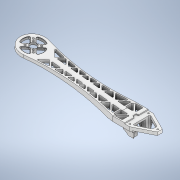
# Autodesk Inventor part: Arm - White
Saved by Autodesk Inventor 2021 (Build 250183000, 183)
## iProperties
Created: 2020-04-25
Part Number: Arm - White
Material: PC/ABS Plastic
Document SubType Name: Modeling
Designer: ljubi
Density: 0.357273 g/cm^3
Appearance: Smooth - White
Author: ljubi
Autodesk Inventor part; units mm, degrees
ref_plane "YZ Plane" through (0, 0, 0) normal (1, 0, 0) x (0, 1, 0)
ref_plane "XZ Plane" through (0, 0, 0) normal (0, 1, 0) x (-1, 0, 0)
ref_plane "XY Plane" through (0, 0, 0) normal (0, 0, 1) x (1, 0, 0)
sketch "Sketch1" plane through (0, 0, 0) normal (0, 1, 0) x (-1, 0, 0)
  line L0 (12, -19) -> (12, 19)
  line L1 (12, 19) -> (0, 19)
  line L2 (0, 19) -> (-30, 4)
  line L3 (-30, 4) -> (-30, -4)
  line L4 (-30, -4) -> (0, -19)
  line L5 (0, -19) -> (12, -19)
  point P0 (0, 0)
  dimension "d0" = 38
  dimension "d1" = 19
  dimension "d2" = 12
  dimension "d3" = 8
  dimension "d4" = 4
  dimension "d5" = 30
  constraints: 12 end point, 2 point on line, 2 vertical alignment, 1 horizontal, 1 parallel, 1 perpendicular, 1 vertical
  measures "d0" distance between parallel lines of L1 L5
  measures "d1" distance from line of L1 point (0, 0)
  measures "d2" distance of L0.end L1.end
  measures "d3" distance of L2.end L3.end
  measures "d4" vertical distance of L2.end point (0, 0)
  measures "d5" distance from line of L3 point (0, 0)
extrude "Extrusion1" add sketch "Sketch1" against normal blind 5
sketch "Sketch2" plane through (0, 0, 0) normal (0, 1, 0) x (1, 0, 0)
  line L0 (0, -19) -> (-12, -19) projected
  line L1 (-12, 19) -> (0, 19) projected
  line L2 (-12, -19) -> (-8, -19)
  line L3 (-8, -19) -> (-8, 19)
  line L4 (-8, 19) -> (-12, 19)
  line L5 (-12, 19) -> (-12, -19)
  point P0 (0, 0)
  dimension "d8" = 8
  constraints: 8 end point, 2 parallel, 1 horizontal, 1 perpendicular, 1 point on line
  measures "d8" distance from line of L3 L1.end
extrude "Extrusion2" add sketch "Sketch2" along normal blind 1.5
sketch "Sketch3" plane through (0, 1.5, 0) normal (0, 1, 0) x (1, 0, 0)
  line L0 (-8, 19) -> (-8, -19) projected
  line L1 (-11.5, -3) -> (-8, -3)
  line L2 (-8, -3) -> (-8, 3)
  line L3 (-8, 3) -> (-11.5, 3)
  line L4 (-11.5, 3) -> (-11.5, -3)
  point P0 (0, 0)
  point P1 (-8, 0)
  dimension "d11" = 6
  dimension "d12" = 3.5
  constraints: 8 end point, 2 midpoint, 2 parallel, 1 horizontal, 1 perpendicular, 1 point on line
  measures "d11" distance between parallel lines of L1 L3
  measures "d12" distance between parallel lines of L4 L0
extrude "Extrusion3" cut sketch "Sketch3" against normal up to surface (1.5 mm away)
fillet "Fillet1" radius 1 4 edges at (-11.5, 0.75, -3) (-11.5, 0.75, 3) (-8, 0.75, 3) (-8, 0.75, -3)
sketch "Sketch4" plane through (0, 0, 0) normal (0, 1, 0) x (1, 0, 0)
  line L0 (30, 4) -> (0, 19) projected
  line L1 (0, -19) -> (30, -4) projected
  line L2 (22, 3.5279) -> (0, 14.5279)
  line L3 (0, -14.5279) -> (22, -3.5279)
  line L4 (22, 3.5279) -> (22, -3.5279)
  line L5 (30, -4) -> (30, 4) projected
  line L6 (0, 14.5279) -> (0, -14.5279)
  point P0 (0, 0)
  dimension "d16" = 4
  dimension "d17" = 4
  dimension "d18" = 8
  constraints: 8 end point, 2 parallel, 2 vertical, 1 point on line
  measures "d16" distance between parallel lines of L1 L3
  measures "d17" distance between parallel lines of L0 L2
  measures "d18" distance between parallel lines of L4 L5
extrude "Extrusion4" cut sketch "Sketch4" against normal through all
fillet "Fillet2" radius 1.5 4 edges at (0, -2.5, -14.5279) (0, -2.5, 14.5279) (22, -2.5, 3.5279) (22, -2.5, -3.5279)
sketch "Sketch5" plane through (-12, -5, -19) normal (-1, 0, 0) x (0, 0, 1)
  line L0 (0, 0) -> (0, 6.5) projected
  line L1 (38, 0) -> (0, 0) projected
  line L2 (38, 6.5) -> (38, 0) projected
  line L3 (0, 6.5) -> (38, 6.5) projected
  point P0 (19, 5)
extrude "Extrusion5" add sketch "Sketch5" along normal blind 15
sketch "Sketch6" plane through (-27, -5, -19) normal (-1, 0, 0) x (0, 0, 1)
  line L0 (0, 0) -> (38, 0)
  line L1 (38, 0) -> (38, -3.5)
  line L2 (38, -3.5) -> (0, -3.5)
  line L3 (0, -3.5) -> (0, 0)
  line L4 (38, 0) -> (38, 6.5) projected
  line L5 (38, 6.5) -> (0, 6.5) projected
  line L6 (0, 6.5) -> (0, 0) projected
  point P0 (19, 5)
  dimension "d24" = 10
  constraints: 8 end point, 2 collinear, 2 parallel, 1 horizontal, 1 perpendicular
  measures "d24" distance between parallel lines of L2 L5
extrude "Extrusion6" add sketch "Sketch6" against normal blind 30 contours L0 L1 L2 L3
sketch "Sketch7" plane through (-8, 0, 19) normal (0, 0, 1) x (1, 0, 0)
  line L0 (11, -8.5) -> (11, -5) projected
  line L1 (11, -8.5) -> (9.2367, -18.5)
  line L2 (9.2367, -18.5) -> (1.2367, -18.5)
  circle A0 centre (-19, -33.9763) radius 25.4763
  line L3 (-19, -8.5) -> (11, -8.5) projected
  line L4 (-19, -8.5) -> (-19, 1.5) projected
  line L5 (0, 1.5) -> (-19, 1.5) projected
  point P0 (8, 0)
  dimension "d27" = 20
  dimension "d28" = 100
  dimension "d29" = 8
  constraints: 4 end point, 1 horizontal, 1 perpendicular, 1 point on line, 3 other
  measures "d27" distance between parallel lines of L2 L5
  measures "d28" angle of L1 L2
  measures "d29" distance of L1.end L2.end
extrude "Extrusion7" add sketch "Sketch7" against normal up to surface (38 mm away) contours L1 L2 A0 L3
sketch "Sketch8" plane through (3, -5, 13.0279) normal (0, 1, 0) x (1, 0, 0)
  line L0 (0, 26.0557) -> (-0.8292, 26.4703) projected
  arc A0 (-0.8292, 26.4703) -> (-3, 25.1287) centre (-1.5, 25.1287) ccw projected
  line L1 (-3, 25.1287) -> (-3, 0.9271) projected
  arc A1 (-3, 0.9271) -> (-0.8292, -0.4146) centre (-1.5, 0.9271) ccw projected
  line L2 (-0.8292, -0.4146) -> (0, 0) projected
  line L3 (0, 26.0557) -> (0, 0) projected
  line L4 (-3, 32.0279) -> (0, 30.5279) projected
  line L5 (0, 32.0279) -> (0, 30.5279) projected
  line L6 (-3, 32.0279) -> (0, 32.0279) projected
  line L7 (0, -4.4721) -> (-3, -5.9721) projected
  line L8 (-3, -5.9721) -> (0, -5.9721) projected
  line L9 (0, -4.4721) -> (0, -5.9721) projected
  point P0 (-3, 13.0279)
extrude "Extrusion8" cut sketch "Sketch8" against normal through all
sketch "Sketch9" plane through (0, 0, 12.1008) normal (1, 0, 0) x (0, 0, -1)
  line L0 (-6.8992, -18.5) -> (31.1008, -18.5) projected
  line L1 (5.6008, -18.5) -> (18.6008, -18.5)
  line L2 (18.6008, -18.5) -> (18.6008, -3)
  line L3 (18.6008, -3) -> (5.6008, -3)
  line L4 (5.6008, -3) -> (5.6008, -18.5)
  line L5 (12.1008, 0) -> (12.1008, -26.1716) construction
  line L6 (16.1008, 0) -> (31.1008, 0) projected
  point P0 (12.1008, -18.5)
  dimension "d34" = 13
  dimension "d35" = 3
  constraints: 10 end point, 2 parallel, 2 point on line, 1 horizontal, 1 midpoint, 1 perpendicular, 1 vertical
  measures "d34" distance between parallel lines of L4 L2
  measures "d35" distance between parallel lines of L6 L3
extrude "Extrusion9" cut sketch "Sketch9" against normal blind 6.5
sketch "Sketch10" plane through (-6.5, 0, 12.1008) normal (1, 0, 0) x (0, 0, -1)
  line L0 (-6.8992, -18.5) -> (31.1008, -18.5) projected
  line L1 (5.6008, -18.5) -> (5.6008, -3) projected
  line L2 (18.6008, -3) -> (18.6008, -18.5) projected
  arc A0 (18.6008, -15) -> (5.6008, -15) centre (12.1008, -15) ccw
  line L3 (-6.8992, 1.5) -> (8.1008, 1.5) projected
  point P0 (12.1008, 0)
  dimension "d38" = 16.5
  constraints: 2 point on circle, 2 point on line, 2 tangent, 1 centre point
  measures "d38" distance from line of A0.centre L3
extrude "Extrusion10" cut sketch "Sketch10" against normal through all
sketch "Sketch11" plane through (-8, 0, 19) normal (0, 0, 1) x (1, 0, 0)
  line L0 (-19, 1.5) -> (-19, -8.5) projected
  line L1 (-19, 1.5) -> (-188.0687, 19.2698)
  line L2 (-188.0687, 19.2698) -> (-188.5914, 14.2972)
  line L3 (0, 1.5) -> (-19, 1.5) projected
  line L4 (-188.5914, 14.2972) -> (-138.8653, 9.0708)
  line L5 (-138.8653, 9.0708) -> (-19, -8.5)
  point P0 (8, 0)
  dimension "d41" = 6
  dimension "d42" = 5
  dimension "d43" = 170
  dimension "d44" = 50
  constraints: 8 end point, 1 parallel, 1 perpendicular
  measures "d41" angle of L1 L3
  measures "d42" distance of L1.end L2.end
  measures "d43" distance of L0.start L1.end
  measures "d44" distance of L2.end L4.end
extrude "Extrusion11" add sketch "Sketch11" against normal up to surface (38 mm away)
sketch "Sketch12" plane through (-196.0687, 19.2698, 19) normal (0.1045285, 0.9945219, 0) x (0.9945219, -0.1045285, 0)
  arc A0 (12.0557, 38) -> (12.0557, 0) centre (21, 19) ccw
  line L0 (197.0089, 6.8992) -> (197.0089, 31.1008) projected
  line L1 (0, 0) -> (0, 38) projected
  line L2 (170, 38) -> (0, 38) projected
  line L3 (170, 0) -> (0, 0) projected
  point P0 (197.0089, 19)
  point P1 (197.0089, 19)
  point P2 (0, 19)
  dimension "d47" = 42
  constraints: 2 point on circle, 2 point on line, 1 centre point, 1 horizontal alignment, 1 midpoint, 1 tangent
  measures "d47" diameter of A0
extrude "Extrusion12" cut sketch "Sketch12" against normal through all
sketch "Sketch13" plane through (-27, 1.5, 19) normal (0.1045285, 0.9945219, 0) x (0.9945219, -0.1045285, 0)
  circle A0 centre (-149, 19) radius 21
  arc A1 (-157.9443, 38) -> (-157.9443, 0) centre (-149, 19) ccw projected
  line L0 (0, 0) -> (-157.9443, 0) projected
  line L1 (0, 38) -> (-157.9443, 38) projected
  point P0 (27.0089, 19)
  point P1 (-140.0557, 38)
  point P2 (-140.0557, 0)
  point P3 (-157.9443, 0)
  constraints: 2 concentric, 1 centre point
extrude "Extrusion13" add sketch "Sketch13" against normal up to surface (5 mm away) contours A0 L1 | L0 A0
sketch "Sketch14" plane through (-27, 1.5, 19) normal (0.1045285, 0.9945219, 0) x (0.9945219, -0.1045285, 0)
  circle A0 centre (-69, -332.0556) radius 339.0556
  arc A1 (-140.0557, 38) -> (-140.0557, 0) centre (-149, 19) ccw projected
  line L0 (-180.4979, 7) -> (84.0441, 7) construction
  line L1 (0, 0) -> (0, 38) projected
  line L2 (0, 0) -> (-140.0557, 0) projected
  point P0 (27.0089, 19)
  point P1 (-137.5403, 0)
  point P2 (-0.4597, 0)
  dimension "d52" = 12
  dimension "d53" = 69
  constraints: 2 end point, 2 tangent, 1 centre point, 1 horizontal
  measures "d52" distance from line of point (27.009, 19) L0
  measures "d53" distance from line of A0.centre L1
extrude "Extrusion14" cut sketch "Sketch14" against normal through all contours L2 A0 picked at (-53.7101, 1.2943)
sketch "Sketch15" plane through (-27, 1.5, 19) normal (0.1045285, 0.9945219, 0) x (0.9945219, -0.1045285, 0)
  circle A0 centre (-69, -332.0556) radius 339.0556
  arc A1 (-0.4597, 0) -> (-137.5403, 0) centre (-69, -332.0556) ccw projected
  line L0 (-137.5403, 0) -> (-140.0557, 0) projected
  arc A2 (-140.0557, 38) -> (-140.0557, 0) centre (-149, 19) ccw projected
  point P0 (27.0089, 19)
  point P1 (-144.3341, -1.4751)
  point P2 (-137.5403, 0)
  constraints: 2 concentric, 1 centre point
extrude "Extrusion15" add sketch "Sketch15" against normal up to surface (5 mm away) contours A2 L0 A0
mirror "Mirror1" about plane through (0, 0, 0) normal (0, 0, 1) of "Extrusion14", "Extrusion15"
sketch "Sketch16" plane through (-27, 1.5, 19) normal (0.1045285, 0.9945219, 0) x (0.9945219, -0.1045285, 0)
  circle A0 centre (-149, 19) radius 5.5
  arc A1 (-144.3341, 39.4751) -> (-144.3341, -1.4751) centre (-149, 19) ccw projected
  point P0 (27.0089, 19)
  dimension "d58" = 11
  constraints: 1 centre point, 1 concentric
  measures "d58" diameter of A0
extrude "Extrusion16" cut sketch "Sketch16" against normal through all
sketch "Sketch17" plane through (-27, 1.5, 19) normal (0.1045285, 0.9945219, 0) x (0.9945219, -0.1045285, 0)
  circle A0 centre (-149, 19) radius 5.5 projected
  line L0 (-149, 19) -> (-171.99, -3.99) construction
  line L1 (-149, 19) -> (-149, -8.9855) construction
  line L2 (-149, 19) -> (-175.0574, 45.0574) construction
  line L3 (-161.209, 12.0943) -> (-155.364, 17.9393)
  line L4 (-161.209, 25.9057) -> (-155.364, 20.0607)
  arc A1 (-144.3341, 39.4751) -> (-144.3341, -1.4751) centre (-149, 19) ccw projected
  arc A2 (-163.6424, 25.4497) -> (-163.6424, 12.5503) centre (-149, 19) ccw
  arc A3 (-155.364, 17.9393) -> (-155.364, 20.0607) centre (-156.4246, 19) ccw
  arc A4 (-161.209, 25.9057) -> (-163.6424, 25.4497) centre (-162.2697, 24.8451) ccw
  arc A5 (-163.6424, 12.5503) -> (-161.209, 12.0943) centre (-162.2697, 13.1549) ccw
  point P0 (27.0089, 19)
  dimension "d61" = 45
  dimension "d62" = 90
  dimension "d63" = 3.75
  dimension "d64" = 3.75
  dimension "d65" = 5
  dimension "d66" = 1.5
  constraints: 10 end point, 8 point on circle, 6 tangent, 4 centre point, 2 equal radius, 2 parallel, 1 vertical
  measures "d61" angle of L1 L0
  measures "d62" angle of L2 L0
  measures "d63" distance between parallel lines of L0 L3
  measures "d64" distance between parallel lines of L2 L4
  measures "d65" radial gap between concentric circles of A1 A2
  measures "d66" radius of A3
extrude "Extrusion17" cut sketch "Sketch17" against normal through all contours A5 A2 A4 L4 A3 L3
pattern_circular "Circular Pattern1" count 4 over 360 about axis through (-175.1838, 17.0747, 0) along (-0.1045285, -0.9945219, 0) of "Extrusion17"
sketch "Sketch18" plane through (-175.7064, 12.1021, 0) normal (-0.1045285, -0.9945219, 0) x (0.9945219, -0.1045285, 0)
  circle A0 centre (0, 0) radius 18
  arc A1 (4.6659, 20.4751) -> (4.6659, -20.4751) centre (0, 0) ccw projected
  point P0 (176.0089, 0)
  dimension "d72" = 36
  constraints: 1 centre point, 1 concentric
  measures "d72" diameter of A0
extrude "Extrusion18" cut sketch "Sketch18" against normal blind 1.5
sketch "Sketch19" plane through (-27, 1.5, 19) normal (0.1045285, 0.9945219, 0) x (0.9945219, -0.1045285, 0)
  line L0 (-161.209, 25.9057) -> (-155.364, 20.0607) projected
  arc A0 (-161.209, 25.9057) -> (-163.6424, 25.4497) centre (-162.2697, 24.8451) ccw projected
  arc A1 (-163.6424, 25.4497) -> (-163.6424, 12.5503) centre (-149, 19) ccw projected
  arc A2 (-163.6424, 12.5503) -> (-161.209, 12.0943) centre (-162.2697, 13.1549) ccw projected
  line L1 (-155.364, 17.9393) -> (-161.209, 12.0943) projected
  arc A3 (-155.364, 17.9393) -> (-155.364, 20.0607) centre (-156.4246, 19) ccw projected
  line L2 (-154.8336, 20.591) -> (-160.6787, 26.4361)
  arc A4 (-160.6787, 26.4361) -> (-164.3288, 25.7521) centre (-162.2697, 24.8451) ccw
  arc A5 (-164.3288, 25.7521) -> (-164.3288, 12.2479) centre (-149, 19) ccw
  arc A6 (-164.3288, 12.2479) -> (-160.6787, 11.5639) centre (-162.2697, 13.1549) ccw
  line L3 (-160.6787, 11.5639) -> (-154.8336, 17.409)
  arc A7 (-154.8336, 17.409) -> (-154.8336, 20.591) centre (-156.4246, 19) ccw
  point P0 (27.0089, 19)
  dimension "d75" = 0.75
  constraints: 8 point on circle, 4 centre point, 4 end point, 5 other
  measures "d75" distance between parallel lines of L2 L0
extrude "Extrusion19" cut sketch "Sketch19" against normal blind 0.5 contours L0 A3 L1 A2 A1 A0 | A7 L3 A6 A5 A4 L2
pattern_circular "Circular Pattern2" count 4 over 360 about axis through (-175.1838, 17.0747, 0) along (-0.1045285, -0.9945219, 0) of "Extrusion19"
sketch "Sketch20" plane through (-175.5496, 13.5939, 0) normal (-0.1045285, -0.9945219, 0) x (0.9945219, -0.1045285, 0)
  line L0 (-6.9057, 12.209) -> (-1.0607, 6.364) projected
  circle A0 centre (0, 0) radius 8 construction
  circle A1 centre (0, 0) radius 9.5 construction
  line L1 (0, 0) -> (-6.7175, 6.7175) construction
  circle A2 centre (-6.7175, 6.7175) radius 1.65
  circle A3 centre (6.7175, -6.7175) radius 1.65
  line L2 (0, 0) -> (6.7175, 6.7175) construction
  circle A4 centre (5.6569, 5.6569) radius 1.65
  circle A5 centre (-5.6569, -5.6569) radius 1.65
  circle A6 centre (0, 0) radius 12.5 construction
  circle A7 centre (8.8388, 8.8388) radius 1.65
  circle A8 centre (-8.8388, -8.8388) radius 1.65
  point P0 (176.0089, 0)
  dimension "d81" = 19
  dimension "d82" = 16
  dimension "d84" = 3.3
  dimension "d85" = 4.5
  constraints: 9 centre point, 7 point on circle, 5 equal radius, 5 point on line, 4 coincident, 4 end point, 1 parallel, 1 perpendicular
  measures "d81" diameter of A1
  measures "d82" diameter of A0
  measures "d84" diameter of A2
  measures "d85" radial gap between concentric circles of A6 A0
extrude "Extrusion20" cut sketch "Sketch20" against normal through all
sketch "Sketch21" plane through (-27, 1.5, 19) normal (0.1045285, 0.9945219, 0) x (0.9945219, -0.1045285, 0)
  line L0 (75.0561, 23) -> (-199.3554, 23)
  arc A0 (-144.3341, 39.4751) -> (-0.4597, 38) centre (-69, 370.0556) ccw projected
  arc A1 (-144.7784, 37.5251) -> (-0.0554, 36.0413) centre (-69, 370.0556) ccw
  line L1 (-69, 370.0556) -> (-69, -89.5128) construction
  line L2 (-69, 29) -> (-75, 23)
  line L3 (-71.8168, 29.0116) -> (-77.8284, 23)
  line L4 (-77.8284, 23) -> (-84.1658, 29.3374)
  line L5 (-80.6569, 23) -> (-87.1396, 29.4827)
  line L6 (-93.6223, 23) -> (-87.1396, 29.4827)
  line L7 (-96.4507, 23) -> (-89.815, 29.6358)
  line L8 (-96.4507, 23) -> (-104.2804, 30.8297)
  line L9 (-99.2792, 23) -> (-107.4539, 31.1748)
  line L10 (-107.4539, 31.1748) -> (-115.6287, 23)
  line L11 (-109.9855, 31.4716) -> (-118.4571, 23)
  line L12 (-118.4571, 23) -> (-129.947, 34.4898)
  line L13 (-69, 29) -> (-63, 23)
  line L14 (-66.1832, 29.0116) -> (-60.1716, 23)
  line L15 (-60.1716, 23) -> (-53.8342, 29.3374)
  line L16 (-57.3431, 23) -> (-50.8604, 29.4827)
  line L17 (-50.8604, 29.4827) -> (-44.3777, 23)
  line L18 (-48.185, 29.6358) -> (-41.5493, 23)
  line L19 (-41.5493, 23) -> (-33.7196, 30.8297)
  line L20 (-38.7208, 23) -> (-30.5461, 31.1748)
  line L21 (-30.5461, 31.1748) -> (-22.3713, 23)
  line L22 (-28.0145, 31.4716) -> (-19.5429, 23)
  line L23 (-19.5429, 23) -> (-8.053, 34.4898)
  point P0 (27.0089, 19)
  dimension "d88" = 4
  dimension "d89" = 2
  dimension "d90" = 45
  dimension "d91" = 2
  dimension "d92" = 45
  dimension "d93" = 2
  dimension "d94" = 45
  dimension "d95" = 2
  dimension "d96" = 45
  dimension "d97" = 2
  dimension "d98" = 45
  dimension "d99" = 2
  dimension "d100" = 45
  dimension "d101" = 45
  dimension "d102" = 2
  dimension "d103" = 45
  dimension "d104" = 2
  dimension "d105" = 45
  dimension "d106" = 2
  dimension "d107" = 45
  dimension "d108" = 2
  dimension "d109" = 45
  dimension "d110" = 2
  dimension "d111" = 45
  constraints: 46 end point, 12 point on line, 10 parallel, 1 vertical, 51 other
  measures "d90" angle of L1 L2
  measures "d91" distance between parallel lines of L2 L3
  measures "d92" angle of L1 L4
  measures "d93" distance between parallel lines of L5 L4
  measures "d94" angle of L1 L6
  measures "d95" distance between parallel lines of L7 L6
  measures "d96" angle of L1 L8
  measures "d97" distance between parallel lines of L8 L9
  measures "d98" angle of L1 L10
  measures "d99" distance between parallel lines of L11 L10
  measures "d100" angle of L1 L12
  measures "d101" angle of L1 L13
  measures "d102" distance between parallel lines of L14 L13
  measures "d103" angle of L1 L15
  measures "d104" distance between parallel lines of L16 L15
  measures "d105" angle of L17 L1
  measures "d106" distance between parallel lines of L18 L17
  measures "d107" angle of L1 L19
  measures "d108" distance between parallel lines of L19 L20
  measures "d109" angle of L1 L21
  measures "d110" distance between parallel lines of L22 L21
  measures "d111" angle of L1 L23
extrude "Extrusion21" cut sketch "Sketch21" against normal through all contours L22 A1 L23 | L0 L20 L21 | L18 A1 L19 | L0 L16 L17 | L14 A1 L15 | L0 L2 L13 | L4 A1 L3 | L0 L6 L5 | L8 A1 L7 | L0 L10 L9 | L12 A1 L11
fillet "Fillet3" radius 1 32 edges at (-156.4964, 12.5969, -15.4898) (-136.6657, 10.3069, -12.4716) (-134.1534, 9.9908, -12.1748) (-142.2659, 11.0114, -4) (-126.0409, 8.9702, -4) (-123.234, 8.6171, -4) (-116.6487, 7.7887, -10.6358) (-131.0041, 9.5946, -11.8297) (-120.4271, 8.264, -4) (-107.5603, 6.6454, -4) (-113.9937, 7.4547, -10.4827) (-111.0425, 7.0834, -10.3374) (-104.7534, 6.2923, -4) (-98.7876, 5.5417, -10.0116) (-101.9465, 5.9391, -4) (-90.0379, 4.441, -4) (-95.9922, 5.1901, -10) (-93.1969, 4.8384, -10.0116) (-87.231, 4.0879, -4) (-80.9419, 3.2967, -10.3374) (-84.4241, 3.7348, -4) (-71.5574, 2.1161, -4) (-77.9907, 2.9255, -10.4827) (-68.7505, 1.763, -4) (-75.3357, 2.5915, -10.6358) (-60.9804, 0.7855, -11.8297) (-57.831, 0.3893, -12.1748) (-65.9436, 1.4099, -4) (-49.7185, -0.6312, -4) (-55.3187, 0.0733, -12.4716) (-46.9116, -0.9843, -4) (-35.5093, -2.4188, -15.4898)
mirror "Mirror2" about plane through (0, 0, 0) normal (0, 0, 1) of "Extrusion21", "Fillet3"
sketch "Sketch22" plane through (-27, 1.5, 19) normal (0.1045285, 0.9945219, 0) x (0.9945219, -0.1045285, 0)
  arc A0 (-0.4597, 0) -> (-144.3341, -1.4751) centre (-69, -332.0556) ccw projected
  arc A1 (-144.3341, 39.4751) -> (-0.4597, 38) centre (-69, 370.0556) ccw projected
  line L0 (-10.2976, 32.2453) -> (-18.8357, 23.7071) projected
  line L1 (-18.8357, 14.2929) -> (-10.2976, 5.7547) projected
  line L2 (-16.7144, 15) -> (-4.5741, 2.8596)
  line L3 (-4.5741, 35.1404) -> (-16.7144, 23)
  arc A2 (-0.0554, 1.9587) -> (-144.7784, 0.4749) centre (-69, -332.0556) ccw
  arc A3 (-144.7784, 37.5251) -> (-0.0554, 36.0413) centre (-69, 370.0556) ccw
  line L4 (-4.5741, 15) -> (-16.7144, 15)
  line L5 (-4.5741, 23) -> (-16.7144, 23)
  line L6 (-24.7855, 23) -> (-36.3066, 23) projected
  line L7 (-36.3066, 15) -> (-24.7855, 15) projected
  line L8 (-4.5741, 2.8596) -> (-4.5741, 15)
  line L9 (-4.5741, 35.1404) -> (-4.5741, 23)
  point P0 (27.0089, 19)
  dimension "d115" = 2
  dimension "d116" = 2
  dimension "d117" = 2
  dimension "d118" = 2
  constraints: 12 end point, 6 point on circle, 2 centre point, 2 collinear, 2 horizontal, 2 parallel, 2 vertical
  measures "d115" radial gap between concentric circles of A0 A2
  measures "d116" radial gap between concentric circles of A1 A3
  measures "d117" distance between parallel lines of L0 L3
  measures "d118" distance between parallel lines of L1 L2
extrude "Extrusion22" cut sketch "Sketch22" against normal through all both and the other way through all
fillet "Fillet4" radius 1 6 edges at (-44.1047, -1.3374, -4) (-32.0568, -2.8531, -4) (-32.0568, -2.8531, -16.1404) (-44.1047, -1.3374, 4) (-32.0568, -2.8531, 4) (-32.0568, -2.8531, 16.1404)
sketch "Sketch23" plane through (0, 1.5, 0) normal (0, 1, 0) x (1, 0, 0)
  line L0 (-31.549, -5) -> (-31.549, -13.7261) projected
  line L1 (-31.549, 13.7261) -> (-31.549, 5) projected
  line L2 (-29.549, -4) -> (-29.549, -16.5754)
  ellipse E0 centre (-95.622, -351.0556) end of major axis (-95.622, -690.1111) minor radius 337.1982 (-27.4571, -19) -> (-170.5434, -20.4751) ccw projected
  line L3 (-41.2219, -4) -> (-32.5435, -4) projected
  line L4 (-8, -19) -> (-27, -19) projected
  ellipse E1 centre (-95.622, -351.0556) end of major axis (-95.622, -692.0696) minor radius 339.1571 (-27.4571, -17) -> (-170.9808, -18.566) ccw
  line L5 (-8, -17) -> (-27.1452, -17)
  line L6 (-12.8545, -4) -> (-29.549, -4)
  line L7 (-29.549, -16.5754) -> (-16.9737, -4)
  line L8 (-27.1452, -17) -> (-14.1452, -4)
  line L9 (-14.1452, -4) -> (-14.1452, -17)
  point P0 (0, 0)
  dimension "d122" = 2
  dimension "d123" = 2
  dimension "d124" = 2
  dimension "d125" = 45
  dimension "d126" = 2
  constraints: 12 end point, 9 point on line, 3 parallel, 1 collinear, 1 horizontal, 1 vertical, 7 other
  measures "d122" distance between parallel lines of L0 L2
  measures "d123" distance between parallel lines of L4 L5
  measures "d124" distance of point (-27.457, -19) point (-27.457, -17)
  measures "d125" angle of L2 L7
  measures "d126" distance between parallel lines of L8 L7
extrude "Extrusion23" cut sketch "Sketch23" against normal through all both and the other way through all
fillet "Fillet5" radius 1 6 edges at (-29.549, -3.1792, 4) (-29.549, -3.1792, 16.5754) (-16.9737, -4.1883, 4) (-14.1452, -4.1883, 4) (-14.1452, -5.2405, 17) (-27.1452, -3.4817, 17)
mirror "Mirror3" about plane through (0, 0, 0) normal (0, 0, 1) of "Extrusion23", "Fillet5"
sketch "Sketch24" plane through (-6.7633, -18.5, 19) normal (0, -1, 0) x (1, 0, 0)
  circle A0 centre (3.2633, -9) radius 1.25
  circle A1 centre (3.2633, -29) radius 1.25
  line L0 (6.7633, -12.5) -> (6.7633, -6.8992) projected
  point P0 (6.7633, -19)
  dimension "d130" = 2.5
  dimension "d131" = 20
  dimension "d132" = 10
  dimension "d133" = 3.5
  constraints: 2 centre point, 1 equal radius, 1 vertical alignment
  measures "d130" diameter of A1
  measures "d131" distance of A1.centre A0.centre
  measures "d132" vertical distance of A1.centre point (6.763, -19)
  measures "d133" distance from line of L0 A0.centre
extrude "Extrusion24" cut sketch "Sketch24" against normal blind 5
sketch "Sketch25" plane through (30, 0, 4) normal (1, 0, 0) x (0, 0, -1)
  line L0 (-15, -18.5) -> (-2.5, -18.5) projected
  line L1 (-10, -18.5) -> (-11.6788, -8.9791)
  line L2 (-17.1975, -6.5) -> (-14.6332, -6.5)
  line L3 (-15, 1.5) -> (0, 1.5) projected
  arc A0 (-11.6788, -8.9791) -> (-14.6332, -6.5) centre (-14.6332, -9.5) ccw
  line L4 (-15, 0) -> (-15, -18.5) projected
  point P0 (4, 0)
  point P1 (-15, -6.5)
  dimension "d136" = 14
  dimension "d137" = 8
  dimension "d138" = 100
  dimension "d139" = 3
  constraints: 4 end point, 2 point on circle, 2 tangent, 1 centre point, 1 horizontal, 1 point on line
  measures "d136" horizontal distance of L1.start point (4, 0)
  measures "d137" distance between parallel lines of L2 L3
  measures "d138" angle of L2 L1
  measures "d139" radius of A0
extrude "Extrusion25" cut sketch "Sketch25" against normal through all
mirror "Mirror4" about plane through (0, 0, 0) normal (0, 0, 1) of "Extrusion25"
sketch "Sketch26" plane through (0, 0, 0) normal (0, 1, 0) x (1, 0, 0)
  circle A0 centre (-3.5, 15) radius 1.25
  circle A1 centre (-3.5, -15) radius 1.25
  circle A2 centre (26.5, 0) radius 1.25
  line L0 (0, -12.1008) -> (0, 12.1008) projected
  line L1 (-8, -19) -> (-8, -4) projected
  point P0 (0, 0)
  point P1 (0, 0)
  dimension "d142" = 2.5
  dimension "d143" = 30
  dimension "d144" = 15
  dimension "d145" = 4.5
  dimension "d146" = 30
  constraints: 3 centre point, 2 equal radius, 1 horizontal alignment, 1 midpoint, 1 vertical alignment
  measures "d142" diameter of A1
  measures "d143" distance of A1.centre A0.centre
  measures "d144" vertical distance of point (0, 0) A1.centre
  measures "d145" distance from line of L1 A1.centre
  measures "d146" horizontal distance of A2.centre A1.centre
extrude "Extrusion26" cut sketch "Sketch26" against normal blind 5
equation "\"d1\" = 0.5 * d0"
equation "\"d4\" = 0.5 * d3"
equation "\"d132\" = 0.5 * d131"
equation "\"d144\" = 0.5 * d143"
body "Solid1"
